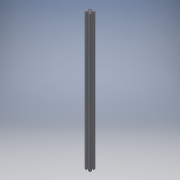
# Autodesk Inventor part: Propile0
Saved by Autodesk Inventor 2019 (Build 230136000, 136)
## iProperties
Created: 2019-04-03
Part Number: Propile0
Material: 알루미늄 6061
Document SubType Name: Modeling
Designer: hinmo
Density: 2.7 g/cm^3
Appearance: 알루미늄 - 평지
Mass: 197.896 g
Surface Area: 1053.21 cm^2
Volume: 73.2946 cm^3
Author: hinmo
Autodesk Inventor part; units mm, degrees
ref_plane "YZ Plane" through (0, 0, 0) normal (1, 0, 0) x (0, 1, 0)
ref_plane "XZ Plane" through (0, 0, 0) normal (0, 1, 0) x (-1, 0, 0)
ref_plane "XY Plane" through (0, 0, 0) normal (0, 0, 1) x (1, 0, 0)
sketch "스케치1" plane through (0, 0, 0) normal (0, 1, 0) x (-1, 0, 0)
  line L0 (9, 10) -> (-9, 10)
  line L1 (-10, 9) -> (-10, -9)
  line L2 (-9, -10) -> (9, -10)
  line L3 (10, -9) -> (10, 9)
  line L4 (10, 10) -> (-10, -10) construction
  line L5 (-10, 10) -> (10, -10) construction
  line L6 (10, 0) -> (-10, 0)
  line L7 (10, 2.65) -> (10, -2.65)
  line L8 (10, -2.65) -> (8.5, -2.65)
  line L9 (8.5, -2.65) -> (8.5, -4.15)
  line L10 (8.5, -4.15) -> (3.3, -4.15)
  line L11 (3.3, 4.15) -> (8.5, 4.15)
  line L12 (8.5, 4.15) -> (8.5, 2.65)
  line L13 (8.5, 2.65) -> (10, 2.65)
  line L14 (8.5, 4.15) -> (4.9, 4.15)
  line L15 (4.9, 4.15) -> (4.9, -4.15)
  arc A0 (4.9, 4.15) -> (4.9, -4.15) centre (9.482, 0) ccw
  line L16 (2.65, -10) -> (-2.65, -10)
  line L17 (-2.65, -10) -> (-2.65, -8.5)
  line L18 (-2.65, -8.5) -> (-4.15, -8.5)
  line L19 (-4.15, -8.5) -> (-4.15, -3.3)
  line L20 (4.15, -3.3) -> (4.15, -8.5)
  line L21 (4.15, -8.5) -> (2.65, -8.5)
  line L22 (2.65, -8.5) -> (2.65, -10)
  line L23 (4.15, -8.5) -> (4.15, -4.9)
  line L24 (4.15, -4.9) -> (-4.15, -4.9)
  arc A1 (4.15, -4.9) -> (-4.15, -4.9) centre (0, -9.482) ccw
  line L25 (-10, -2.65) -> (-10, 2.65)
  line L26 (-10, 2.65) -> (-8.5, 2.65)
  line L27 (-8.5, 2.65) -> (-8.5, 4.15)
  line L28 (-8.5, 4.15) -> (-3.3, 4.15)
  line L29 (-3.3, -4.15) -> (-8.5, -4.15)
  line L30 (-8.5, -4.15) -> (-8.5, -2.65)
  line L31 (-8.5, -2.65) -> (-10, -2.65)
  line L32 (-8.5, -4.15) -> (-4.9, -4.15)
  line L33 (-4.9, -4.15) -> (-4.9, 4.15)
  arc A2 (-4.9, -4.15) -> (-4.9, 4.15) centre (-9.482, 0) ccw
  line L34 (4.15, 8.5) -> (4.15, 3.3)
  line L35 (2.65, 8.5) -> (4.15, 8.5)
  line L36 (2.65, 10) -> (2.65, 8.5)
  line L37 (-2.65, 10) -> (2.65, 10)
  line L38 (-2.65, 8.5) -> (-2.65, 10)
  line L39 (-4.15, 4.9) -> (4.15, 4.9)
  arc A3 (-4.15, 4.9) -> (4.15, 4.9) centre (0, 9.482) ccw
  line L40 (-4.15, 8.5) -> (-4.15, 4.9)
  line L41 (-4.15, 8.5) -> (-2.65, 8.5)
  line L42 (-4.15, 3.3) -> (-4.15, 8.5)
  line L43 (0, 10) -> (7, 10)
  line L44 (7, 10) -> (7, 7)
  circle A4 centre (7, 7) radius 2
  circle A5 centre (0, 0) radius 2.15
  line L45 (7, 7) -> (-7, 7)
  line L46 (-7, 7) -> (-7, -7)
  line L47 (-7, -7) -> (7, -7)
  circle A6 centre (7, -7) radius 2
  circle A7 centre (-7, -7) radius 2
  circle A8 centre (-7, 7) radius 2
  arc A9 (10, 9) -> (9, 10) centre (9, 9) ccw
  arc A10 (-9, 10) -> (-10, 9) centre (-9, 9) ccw
  arc A11 (-10, -9) -> (-9, -10) centre (-9, -9) ccw
  arc A12 (9, -10) -> (10, -9) centre (9, -9) ccw
  point P0 (0, -10)
  point P1 (-10, 0)
  point P2 (0, 10)
  point P3 (-3.3, 4.15)
  point P4 (3.3, 4.15)
  dimension "d0" = 20
  dimension "d1" = 20
  dimension "d2" = 2.65
  dimension "d3" = 5.3
  dimension "d4" = 1.5
  dimension "d5" = 1.5
  dimension "d6" = 5.2
  dimension "d8" = 8.3
  dimension "d9" = 5.2
  dimension "d10" = 1.5
  dimension "d11" = 3.6
  dimension "d12" = 2.65
  dimension "d13" = 5.3
  dimension "d14" = 1.5
  dimension "d15" = 1.5
  dimension "d16" = 5.2
  dimension "d17" = 8.3
  dimension "d18" = 5.2
  dimension "d19" = 1.5
  dimension "d20" = 3.6
  dimension "d21" = 2.65
  dimension "d22" = 5.3
  dimension "d23" = 1.5
  dimension "d24" = 1.5
  dimension "d25" = 5.2
  dimension "d26" = 8.3
  dimension "d27" = 5.2
  dimension "d28" = 1.5
  dimension "d29" = 3.6
  dimension "d30" = 2.65
  dimension "d31" = 5.3
  dimension "d32" = 1.5
  dimension "d33" = 1.5
  dimension "d34" = 5.2
  dimension "d35" = 8.3
  dimension "d36" = 5.2
  dimension "d37" = 1.5
  dimension "d38" = 3.6
  dimension "d39" = 7
  dimension "d40" = 4
  dimension "d41" = 4.3
  dimension "d42" = 4
  dimension "d43" = 4
  dimension "d44" = 4
  dimension "d45" = 1
  constraints: 96 end point, 24 perpendicular, 23 point on line, 16 point on circle, 13 centre point, 8 tangent, 5 coincident, 4 midpoint, 3 equal radius, 3 horizontal, 2 parallel
  measures "d0" distance of L5.end L4.end
  measures "d1" distance of L4.end L5.start
  measures "d2" distance of L6.start L7.start
  measures "d3" distance of L7.start L7.end
  measures "d4" distance of L7.end L8.end
  measures "d5" distance of L8.end L9.end
  measures "d6" distance of L9.end L10.end
  measures "d8" distance of L10.end L11.start
  measures "d9" distance of L11.start L11.end
  measures "d10" distance of L11.end L12.end
  measures "d11" distance of L11.end L14.end
  measures "d12" distance of point (0, -10) L22.end
  measures "d13" distance of L22.end L16.end
  measures "d14" distance of L16.end L18.start
  measures "d15" distance of L18.start L18.end
  measures "d16" distance of L18.end L19.end
  measures "d17" distance of L19.end L20.start
  measures "d18" distance of L20.start L20.end
  measures "d19" distance of L20.end L21.end
  measures "d20" distance of L20.end L24.start
  measures "d21" distance of point (-10, 0) L25.start
  measures "d22" distance of L25.start L26.start
  measures "d23" distance of L26.start L27.start
  measures "d24" distance of L27.start L28.start
  measures "d25" distance of L28.start L28.end
  measures "d26" distance of L28.end L29.start
  measures "d27" distance of L29.start L32.start
  measures "d28" distance of L32.start L31.start
  measures "d29" distance of L32.start L33.start
  measures "d30" distance of L43.start L38.end
  measures "d31" distance of L38.end L37.end
  measures "d32" distance of L37.end L35.start
  measures "d33" distance of L35.start L35.end
  measures "d34" distance of L35.end L34.end
  measures "d35" distance of L34.end L42.start
  measures "d36" distance of L42.start L42.end
  measures "d37" distance of L42.end L41.end
  measures "d38" distance of L42.end L40.end
  measures "d39" distance of L43.start L43.end
  measures "d40" diameter of A4
  measures "d41" diameter of A5
  measures "d42" diameter of A6
  measures "d43" diameter of A7
  measures "d44" diameter of A8
  measures "d45" radius of A9
extrude "돌출1" add sketch "스케치1" along normal blind 500 contours A9 L3 L13 L12 L11 L34 L45 A4 L44 L0 | L44 A4 L45 L34 L35 L36 L0 | L38 L41 L40 L45 A8 L46 L28 L27 L26 L1 A10 L0 | L3 A12 L2 L22 L21 L20 L10 L9 L8 | L34 L11 A0 L6 A5 A2 L28 L42 A3 | L40 L42 L28 L46 A8 L45 | A0 L10 L20 A1 L19 L29 A2 L6 A5 | L2 A11 L1 L31 L30 L29 L46 A7 L47 L19 L18 L17 | L19 L47 A7 L46 L29
